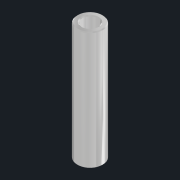
# Autodesk Inventor part: MainHilt
Saved by Autodesk Inventor 2022.2 (Build 262287000, 287)
## iProperties
Manager: Robert Michael Lacey
Company: RM Lacey Machine
Created: 2022-01-30
Part Number: MainHilt
Material: Aluminum 6061
Document SubType Name: Modeling
Designer: Michael Lacey
Mass: 329.845 g
Surface Area: 439.999 cm^2
Volume: 122.165 cm^3
Density: 2.7 g/cm^3
Appearance: Aluminum - Flat
Stock Number: 1
Author: Michael Lacey
Title: Main Hilt
Subject: LightSaber Prop
Autodesk Inventor part; units mm, degrees
ref_plane "YZ Plane" through (0, 0, 0) normal (1, 0, 0) x (0, 1, 0)
ref_plane "XZ Plane" through (0, 0, 0) normal (0, 1, 0) x (-1, 0, 0)
ref_plane "XY Plane" through (0, 0, 0) normal (0, 0, 1) x (1, 0, 0)
sketch "Sketch1" plane through (0, 0, 0) normal (0, 1, 0) x (-1, 0, 0)
  line L0 (12.6023, 12.4715) -> (19.7143, 12.4715)
  line L1 (19.7143, 12.4715) -> (19.7143, -101.8285)
  line L2 (12.6023, 37.8715) -> (15.7773, 37.8715)
  line L3 (15.7773, 37.8715) -> (15.7773, 88.6715)
  line L4 (12.6023, 37.8715) -> (12.6023, 12.4715)
  line L5 (3.0773, 143.0573) -> (3.0773, -154.5984) construction
  line L6 (15.7773, 88.6715) -> (23.7148, 88.6715)
  line L7 (23.7148, 88.6715) -> (23.7148, -101.8285)
  line L8 (23.7148, -101.8285) -> (19.7143, -101.8285)
  point P0 (0, 0)
  dimension "d1" = 114.3
  dimension "d3" = 50.8
  dimension "d5" = 3.175
  dimension "d6" = 20.6375
  dimension "d10" = 12.7
  dimension "d14" = 16.637
  constraints: 18 end point, 4 perpendicular, 3 horizontal, 1 vertical
  measures "d1" distance of L0.end L1.end
  measures "d3" distance of L3.end L2.end
  measures "d5" distance between parallel lines of L3 L4
  measures "d6" distance between parallel lines of L5 L7
  measures "d10" distance between parallel lines of L5 L3
  measures "d14" distance from line of L5 L1.end
revolve "Revolution1" add sketch "Sketch1" angle 360 about axis through (-3.0773, 0, 143.0573) along (0, 0, -1)
chamfer "Chamfer1" distance 1.27 angle 45 4 edges at (17.5602, 0, -101.8285) (17.5602, 0, 88.6715) (9.6227, 0, 88.6715) (13.5597, 0, -101.8285)
thread "Thread1" size "1 5/16-18 UNEF" class "2B" standard "ANSI Unified Screw Threads" length 25.4
body "Solid1"
